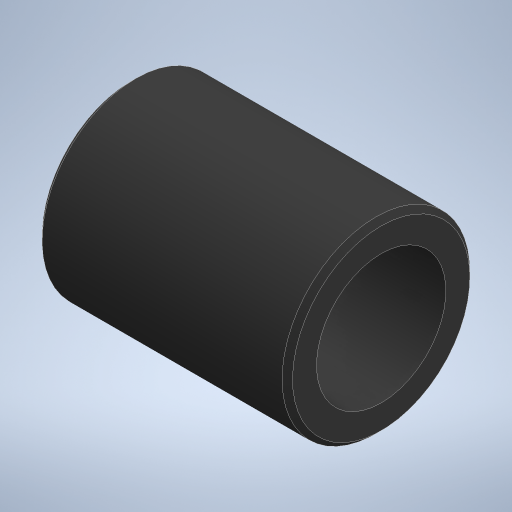
# Autodesk Inventor part: Z-screw Bump Stop
Saved by Autodesk Inventor 2024 (Build 280153000, 153)
## iProperties
Created: 2025-01-01
Part Number: Z-screw Bump Stop
Material: Rubber, Silicone
Document SubType Name: Modeling
Designer: Ishaan
Density: 1.25 g/cm^3
Appearance: Rubber - Black
Author: Ishaan
Autodesk Inventor part; units mm, degrees
ref_plane "YZ Plane" through (0, 0, 0) normal (1, 0, 0) x (0, 1, 0)
ref_plane "XZ Plane" through (0, 0, 0) normal (0, 1, 0) x (-1, 0, 0)
ref_plane "XY Plane" through (0, 0, 0) normal (0, 0, 1) x (1, 0, 0)
sketch "Sketch1" plane through (0, 0, 0) normal (1, 0, 0) x (0, 1, 0)
  circle A0 centre (0, 0) radius 6.2
  circle A1 centre (0, 0) radius 9
  dimension "d0" = 12.4
  dimension "d1" = 18
  constraints: 2 centre point, 2 coincident
  measures "d0" diameter of A0
  measures "d1" diameter of A1
extrude "Extrusion1" add sketch "Sketch1" along normal blind 24
chamfer "Chamfer1" distance 0.5 angle 45 2 edges at (0, -9, 0) (24, -9, 0)
body "Solid1"
